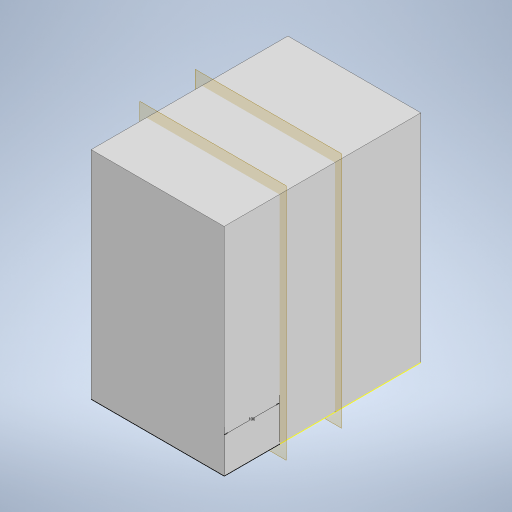
# Autodesk Inventor part: pump support
Saved by Autodesk Inventor 2023 (Build 270158000, 158)
## iProperties
Created: 2022-10-05
Part Number: pump support
Material: Generic
Document SubType Name: Modeling
Designer: station
Density: 1 g/cm^3
Appearance: Default
Mass: 33228 g
Surface Area: 6345 cm^2
Volume: 33228 cm^3
Author: station
Autodesk Inventor part; units mm, degrees
ref_plane "YZ Plane" through (0, 0, 0) normal (1, 0, 0) x (0, 1, 0)
ref_plane "XZ Plane" through (0, 0, 0) normal (0, 1, 0) x (-1, 0, 0)
ref_plane "XY Plane" through (0, 0, 0) normal (0, 0, 1) x (1, 0, 0)
sketch "Sketch1" plane through (0, 0, 0) normal (0, 1, 0) x (-1, 0, 0)
  line L0 (0, 0) -> (-240, 0)
  line L1 (-240, 0) -> (-240, -355)
  line L2 (-240, -355) -> (0, -355)
  line L3 (0, -355) -> (0, 0)
  dimension "d0" = 240
  dimension "d1" = 355
  constraints: 8 end point, 2 parallel, 1 horizontal, 1 perpendicular
  measures "d0" distance of L2.end L1.end
  measures "d1" distance of L1.end L0.end
extrude "Extrusion1" add sketch "Sketch1" along normal blind 390
sketch "Sketch7" plane through (0, 0, 0) normal (0, 0, 1) x (1, 0, 0)
  line L0 (240, 0) -> (0, 0) projected
  line L1 (0, 0) -> (240, 0)
  constraints: 2 end point, 1 collinear
sketch "Sketch8" plane through (240, 0, 0) normal (1, 0, 0) x (0, 0, -1)
  line L0 (0, 0) -> (355, 0) projected
  line L1 (0, 0) -> (100, 0)
  dimension "d8" = 100
  constraints: 2 end point, 1 point on line
  measures "d8" distance of L0.start L1.end
ref_plane "Work Plane1" through (0, 0, -100) normal (0, 0, 1) x (1, 0, 0)
sketch "Sketch9" plane through (0, 0, -100) normal (0, 0, 1) x (1, 0, 0)
  line L0 (240, 0) -> (0, 0) projected
  line L1 (0, 0) -> (240, 0)
  constraints: 2 end point, 1 horizontal
ref_plane "Work Plane3" through (0, 0, -200) normal (0, 0, 1) x (1, 0, 0)
sketch "Sketch10" plane through (0, 0, -200) normal (0, 0, 1) x (1, 0, 0)
  line L0 (240, 0) -> (0, 0) projected
  line L1 (0, 0) -> (240, 0)
  constraints: 2 end point, 1 collinear
body "Solid1"
